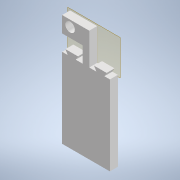
# Autodesk Inventor part: jaws
Saved by Autodesk Inventor 2020 (Build 240168000, 168)
## iProperties
Created: 2020-07-02
Part Number: jaws
Material: Generic
Document SubType Name: Modeling
Designer: Ashiqrahman
Density: 1 g/cm^3
Appearance: Default
Author: Ashiqrahman
Autodesk Inventor part; units mm, degrees
ref_plane "YZ Plane" through (0, 0, 0) normal (1, 0, 0) x (0, 1, 0)
ref_plane "XZ Plane" through (0, 0, 0) normal (0, 1, 0) x (-1, 0, 0)
ref_plane "Work Plane1" through (-60.0293, 37.0443, 146.7859) normal (0, 0, 1) x (1, 0, 0)
sketch "Sketch1" plane through (-60.0293, 37.0443, 146.7859) normal (0, 0, 1) x (1, 0, 0)
  line L0 (55.8868, 5) -> (53, 0) projected
  line L1 (53, 0) -> (60, 0) projected
  line L2 (60, 0) -> (60, 10) projected
  line L3 (20, 10) -> (60, 10) projected
  line L4 (20, 10) -> (20, 40) projected
  line L5 (0, 40) -> (20, 40) projected
  line L6 (0, 0) -> (0, 40) projected
  line L7 (0, 0) -> (7, 0) projected
  line L8 (7, 0) -> (4.1132, 5) projected
  line L9 (4.1132, 5) -> (19.8868, 5) projected
  line L10 (19.8868, 5) -> (17, 0) projected
  line L11 (17, 0) -> (43, 0) projected
  line L12 (43, 0) -> (40.1132, 5) projected
  line L13 (40.1132, 5) -> (55.8868, 5) projected
  circle A0 centre (10, 32) radius 6 projected
  line L14 (0, 0) -> (60, 0)
  line L15 (60, 0) -> (60, -100)
  line L16 (60, -100) -> (0, -100)
  line L17 (0, -100) -> (0, 0)
  point P0 (60.0293, -37.0443)
  dimension "d0" = 60
  dimension "d1" = 100
  constraints: 8 end point, 2 parallel, 1 horizontal, 1 perpendicular
  measures "d0" distance of L15.end L16.end
  measures "d1" distance of L14.end L15.end
extrude "Extrusion1" add sketch "Sketch1" along normal blind 10 contours L0 L14 L12 L13 | L1 L15 L16 L17 L7 L14 L11 | L14 L8 L9 L10
sketch "Sketch2" plane through (-43.0293, 37.0443, 146.7859) normal (0, 1, 0) x (1, 0, 0)
  line L0 (17, -10) -> (9, -10)
  line L1 (9, -10) -> (9, 0)
  line L2 (9, 0) -> (17, 0)
  line L3 (17, 0) -> (17, -10)
  line L4 (17, -10) -> (9, 0) construction
  line L5 (9, -10) -> (17, 0) construction
  line L6 (55.0352, 0) -> (-29.0059, 0) projected
  line L7 (43, 0) -> (43, -10) projected
  point P0 (43.0293, 146.7859)
  point P1 (13, -5)
  dimension "d4" = 8
  dimension "d5" = 10
  dimension "d6" = 0
  dimension "d9" = 30
  constraints: 12 end point, 2 midpoint, 2 parallel, 1 horizontal, 1 perpendicular
  measures "d4" distance of L1.end L2.end
  measures "d5" distance of L0.end L1.end
  measures "d6" distance between parallel lines of L6 L2
  measures "d9" distance from line of L7 point (13, -5)
extrude "Extrusion2" add sketch "Sketch2" along normal up to surface (40 mm away)
sketch "Sketch3" plane through (-34.0293, 37.0443, 146.7859) normal (-1, 0, 0) x (0, 0, 1)
  line L0 (10, 40) -> (0, 40) projected
  line L1 (0, 0) -> (0, 40) projected
  line L2 (10, 0) -> (0, 0) projected
  line L3 (10, 0) -> (10, 40) projected
  line L4 (0, 0) -> (0, 40) projected
  line L5 (0, 20) -> (10, 20)
  point P0 (-146.7859, -37.0443)
  point P1 (0, 20)
  dimension "d10" = 20
  constraints: 2 end point, 2 midpoint, 1 horizontal
  measures "d10" distance between parallel lines of L5 L0
ref_plane "Work Plane2" through (-60.0293, 37.0443, -153.2141) normal (-1, 0, 0) x (0, 0, 1)
extrude "Extrusion3" add sketch "Sketch3" along normal up to surface (26 mm away) contours L3 L5 L1 L0
sketch "Sketch4" plane through (-60.0293, 37.0443, 156.7859) normal (0, 0, 1) x (1, 0, 0)
  circle A0 centre (10, 32) radius 6 projected
  point P0 (60.0293, -37.0443)
extrude "Extrusion4" cut sketch "Sketch4" against normal through all
thread "Thread1" size "M8x1.25" class "6H" standard "ANSI Metric M Profile" length 140
body "Solid1"
